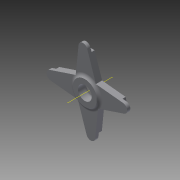
# Autodesk Inventor part: mirror_circular_example
Saved by Autodesk Inventor 2015 (Build 190159000, 159)
## iProperties
Created: 2015-01-28
Part Number: mirror_circular_example
Material: Generic
Document SubType Name: Modeling
Designer: admin
Density: 1 g/cm^3
Appearance: Default
Author: admin
Autodesk Inventor part; units mm, degrees
note: some values were not read from the file. Chosen so that the rebuilt part matches the saved one: copy form of "Circular Pattern1"; copy form of "Circular Pattern2".
ref_plane "YZ Plane" through (0, 0, 0) normal (1, 0, 0) x (0, 1, 0)
ref_plane "XZ Plane" through (0, 0, 0) normal (0, 1, 0) x (-1, 0, 0)
ref_plane "XY Plane" through (0, 0, 0) normal (0, 0, 1) x (1, 0, 0)
sketch "Sketch1" plane through (0, 0, 0) normal (0, 1, 0) x (-1, 0, 0)
  circle A0 centre (0, 0) radius 3.3528
  circle A1 centre (0, 0) radius 5.8383
  dimension "d21" = 11.6765
  dimension "d22" = 6.7056
  constraints: 2 centre point, 2 coincident
  measures "d21" diameter of A1
  measures "d22" diameter of A0
extrude "Extrusion1" add sketch "Sketch1" along normal mid plane 5
sketch "Sketch2" plane through (0, 0, 0) normal (0, 1, 0) x (-1, 0, 0)
  line L0 (5.5433, -1.8324) -> (0.1869, -18.0363)
  arc A0 (-4.069, -17.5723) -> (0.1869, -18.0363) centre (-1.8914, -17.3493) ccw
  line L1 (-4.069, -17.5723) -> (-5.8079, -0.5949)
  circle A1 centre (0, 0) radius 5.8383 projected
  dimension "d23" = 2.1889
  dimension "d24" = 24.14
  constraints: 4 end point, 4 point on circle, 4 tangent, 1 centre point
  measures "d23" radius of A0
  measures "d24" angle of L0 L1
extrude "Extrusion2" add sketch "Sketch2" along normal mid plane 3 contours L0 A0 L1 A1
pattern_circular "Circular Pattern1" count 4 over 360 about axis through (0, -10, 0) along (0, 1, 0) of "Extrusion2" geometry pattern yes
hole "Hole1" at (15.8264, 1.5, -7.5232) direction (0, -1, 0) diameter 1.5 end through all
pattern_circular "Circular Pattern2" count 4 over 360 about axis through (0, -10, 0) along (0, 1, 0) of "Hole1" geometry pattern yes
sketch "Sketch3" plane through (0, 0, 0) normal (1, 0, 0) x (0, 1, 0)
  line L0 (-1.5, -17.5723) -> (-1.5, -4.3565) projected
  line L1 (-1.5, -17.5723) -> (1.5, -17.5723) projected
  line L2 (1.5, -4.3565) -> (1.5, -17.5723) projected
  line L3 (-1.5, -18.0363) -> (1.5, -18.0363) projected
  line L4 (1.5, -17.5723) -> (1.5, -18.0363) projected
  line L5 (-1.5, -17.5723) -> (1.5, -17.5723) projected
  line L6 (-1.5, -18.0363) -> (-1.5, -17.5723) projected
  line L7 (1.5, -19.5382) -> (1.5, -17.5723) projected
  line L8 (-1.5, -19.5382) -> (1.5, -19.5382) projected
  line L9 (-1.5, -17.5723) -> (-1.5, -19.5382) projected
  line L10 (1.5, -7.0294) -> (1.5, -17.5723) projected
  line L11 (1.5, -16.3611) -> (0, -16.3611)
  line L12 (0, -16.3611) -> (0, -20.0305)
  line L13 (0, -20.0305) -> (1.5, -20.0305)
  line L14 (1.5, -20.0305) -> (1.5, -16.3611)
  line L15 (-3.5, 0) -> (3.5, 0) projected
  line L16 (1.5, -4.3565) -> (-1.5, -4.3565) projected
  point P0 (0, 0)
  constraints: 8 end point, 2 parallel, 1 horizontal, 1 perpendicular, 1 point on line
revolve "Revolution1" cut sketch "Sketch3" angle 360 about axis through (0, -10, 0) along (0, 1, 0) contours L12 L11 L2 L1 | L1 L4 L3 L12 | L3 L7 L8 L12 | L8 L14 L13 L12
fillet "Fillet1" radius 2 3 edges at (3.3528, 2.5, 0) (5.8383, 2.5, 0) (5.8383, -1.5, 0)
body "Solid1"
